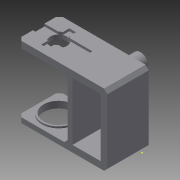
# Autodesk Inventor part: Pinza
Saved by Autodesk Inventor 2015 (Build 190159000, 159)
## iProperties
Created: 2013-10-22
Part Number: Pinza
Material: Genérico
Document SubType Name: Modeling
Designer: Gregorio
Density: 1 g/cm^3
Appearance: Valor por defecto
Author: Gregorio
Autodesk Inventor part; units mm, degrees
ref_plane "YZ Plane" through (0, 0, 0) normal (1, 0, 0) x (0, 1, 0)
ref_plane "XZ Plane" through (0, 0, 0) normal (0, 1, 0) x (-1, 0, 0)
ref_plane "XY Plane" through (0, 0, 0) normal (0, 0, 1) x (1, 0, 0)
sketch "Boceto1" plane through (0, 0, 0) normal (0, 1, 0) x (-1, 0, 0)
  line L0 (0, 0) -> (4, 0)
  line L1 (4, 0) -> (4, 43)
  line L2 (4, 43) -> (0, 43)
  line L3 (0, 43) -> (0, 0)
  line L4 (4, 43) -> (54, 43)
  line L5 (54, 43) -> (54, 39)
  line L6 (54, 39) -> (4, 39)
  line L7 (4, 39) -> (4, 43)
  line L8 (4, 0) -> (54, 0)
  line L9 (54, 0) -> (54, 4)
  line L10 (54, 4) -> (4, 4)
  line L11 (4, 4) -> (4, 0)
  dimension "d4" = 43
  dimension "d5" = 50
  dimension "d6" = 4
  dimension "d7" = 50
  dimension "d8" = 4
  dimension "d54" = 4
  constraints: 24 end point, 6 parallel, 3 horizontal, 3 perpendicular
  measures "d4" distance of L0.end L1.end
  measures "d5" distance of L5.end L6.end
  measures "d6" distance of L4.end L5.end
  measures "d7" distance of L10.end L9.end
  measures "d8" distance of L9.end L8.end
  measures "d54" distance of L1.end L2.end
extrude "Extrusión1" add sketch "Boceto1" along normal blind 25
sketch "Boceto3" plane through (-54, 0, 4) normal (0, 0, 1) x (1, 0, 0)
  line L0 (0, 0) -> (0, 25) projected
  circle A0 centre (12, 12.5) radius 9
  point P0 (54, 0)
  point P1 (0, 12.5)
  dimension "d19" = 18
  dimension "d20" = 12
  constraints: 1 centre point, 1 horizontal alignment, 1 midpoint
  measures "d19" diameter of A0
  measures "d20" distance from line of L0 A0.centre
extrude "Extrusión2" cut sketch "Boceto3" against normal blind 8 and the other way blind 2
sketch "Boceto8" plane through (-54, 0, 43) normal (0, 0, 1) x (1, 0, 0)
  circle A0 centre (12, 12.5) radius 5
  line L0 (0, 0) -> (0, 25) projected
  line L1 (0, 9) -> (0, 16)
  point P0 (0, 12.5)
  dimension "d40" = 10
  dimension "d42" = 12
  constraints: 2 end point, 1 centre point, 1 horizontal alignment, 1 midpoint, 1 point on line
  measures "d40" diameter of A0
  measures "d42" distance from line of L0 A0.centre
extrude "Extrusión7" cut sketch "Boceto8" against normal blind 5
sketch "Boceto9" plane through (-54, 0, 43) normal (0, 0, 1) x (1, 0, 0)
  circle A0 centre (12, 12.5) radius 5 projected
  line L0 (0, 16) -> (29, 16)
  line L1 (29, 16) -> (29, 9)
  line L2 (29, 9) -> (0, 9)
  line L3 (0, 9) -> (0, 16)
  dimension "d44" = 17
  dimension "d45" = 7
  constraints: 8 end point, 2 parallel, 1 horizontal, 1 perpendicular
  measures "d44" distance from line of L1 A0.centre
  measures "d45" distance of L0.end L1.end
sketch "Boceto10" plane through (-54, 0, 43) normal (0, 0, 1) x (1, 0, 0)
  circle A0 centre (12, 12.5) radius 5 projected
  line L0 (0, 0) -> (0, 25) projected
  line L1 (10, 21) -> (14, 21)
  line L2 (14, 21) -> (14, 4)
  line L3 (14, 4) -> (10, 4)
  line L4 (10, 4) -> (10, 21)
  point P0 (10, 12.5)
  point P1 (0, 12.5)
  point P2 (12, 21)
  dimension "d48" = 4
  dimension "d49" = 17
  constraints: 8 end point, 3 midpoint, 2 parallel, 1 horizontal, 1 horizontal alignment, 1 perpendicular, 1 vertical alignment
  measures "d48" distance of L1.start L1.end
  measures "d49" distance of L3.end L1.start
extrude "Extrusión8" cut sketch "Boceto10" against normal blind 1.5 contours L2 A0 L4 | A0 L4 L1 L2 | L2 L3 L4 A0
extrude "Extrusión9" cut sketch "Boceto9" against normal blind 1.5 contours A0 L2 L0 | A0 L0 L1 L2 | A0 L2 L3 L0
chamfer "Chaflán1" distance 2 angle 45 1 edges at (0, 12.5, 0)
chamfer "Chaflán2" distance 2 angle 45 1 edges at (0, 12.5, 43)
sketch "Boceto13" plane through (-54, 0, 4) normal (0, 0, 1) x (1, 0, 0)
  line L0 (0, 25) -> (50, 25) projected
  line L1 (29.9369, 25) -> (49.9369, 25)
  line L2 (49.9369, 25) -> (49.9369, 0)
  line L3 (49.9369, 0) -> (29.9369, 0)
  line L4 (29.9369, 0) -> (29.9369, 25)
  point P0 (54, 0)
  dimension "d80" = 20
  dimension "d81" = 25
  constraints: 8 end point, 2 parallel, 1 horizontal, 1 perpendicular, 1 point on line
  measures "d80" distance of L2.end L3.end
  measures "d81" distance of L3.end L1.start
extrude "Extrusión12" add sketch "Boceto13" along normal blind 5
sketch "Boceto14" plane through (-54, 0, 9) normal (0, 0, 1) x (1, 0, 0)
  line L0 (49.9369, 25) -> (32.9369, 25)
  line L1 (32.9369, 25) -> (32.9369, -5)
  line L2 (32.9369, -5) -> (49.9369, -5)
  line L3 (49.9369, -5) -> (49.9369, 25)
  dimension "d84" = 17
  dimension "d85" = 30
  constraints: 8 end point, 2 parallel, 1 horizontal, 1 perpendicular
  measures "d84" distance of L2.end L1.end
  measures "d85" distance of L1.end L0.end
extrude "Extrusión13" cut sketch "Boceto14" against normal blind 5
sketch "Boceto15" plane through (-4, 0, 4) normal (0, 0, 1) x (1, 0, 0)
  line L0 (0, 25) -> (0, 0) projected
  line L1 (-17.0631, 25) -> (0, 25)
  line L2 (0, 25) -> (0, 21)
  line L3 (0, 21) -> (-17.0631, 21)
  line L4 (-17.0631, 21) -> (-17.0631, 25)
  point P0 (4, 0)
  constraints: 8 end point, 2 parallel, 1 horizontal, 1 perpendicular, 1 point on line
extrude "Extrusión14" add sketch "Boceto15" along normal up to next
sketch "Boceto16" plane through (0, 25, 0) normal (0, 1, 0) x (1, 0, 0)
  circle A0 centre (-13, -15) radius 9
  line L0 (-21.0631, -4) -> (-4, -4) projected
  line L1 (-4, -39) -> (-4, -4) projected
  point P0 (0, 0)
  dimension "d90" = 11
  dimension "d91" = 18
  constraints: 1 centre point, 1 tangent
  measures "d90" distance from line of L0 A0.centre
  measures "d91" diameter of A0
extrude "Extrusión15" cut sketch "Boceto16" against normal blind 5
sketch "Boceto17" plane through (-4, 0, 39) normal (0, 0, -1) x (-1, 0, 0)
  line L0 (0, 0) -> (50, 0) projected
  line L1 (17.0631, 25) -> (20.0631, 25)
  line L2 (20.0631, 25) -> (20.0631, 0)
  line L3 (20.0631, 0) -> (17.0631, 0)
  line L4 (17.0631, 0) -> (17.0631, 25)
  point P0 (-4, 0)
  dimension "d94" = 3
  constraints: 8 end point, 2 parallel, 1 horizontal, 1 perpendicular, 1 point on line
  measures "d94" distance of L2.end L3.end
extrude "Extrusión16" add sketch "Boceto17" along normal up to next
sketch "Boceto18" plane through (0, 25, 0) normal (0, 1, 0) x (1, 0, 0)
  circle A0 centre (-13, -15) radius 9 projected
  line L0 (-54, -43) -> (-2, -43) projected
  circle A1 centre (-13, -35.3) radius 4.75
  point P0 (0, 0)
  dimension "d97" = 9.5
  dimension "d98" = 7.7
  constraints: 1 centre point, 1 vertical alignment
  measures "d97" diameter of A1
  measures "d98" distance from line of L0 A1.centre
extrude "Extrusión17" add sketch "Boceto18" along normal blind 8 contours A1
sketch "Boceto20" plane through (-21.0631, 21, 39) normal (0, -1, 0) x (1, 0, 0)
  arc A0 (17.0631, -24) -> (0, -20.0018) centre (8.0631, -24) ccw projected
  line L0 (0, -20.0018) -> (0, 0) projected
  line L1 (0, 0) -> (17.0631, 0)
  line L2 (17.0631, 0) -> (17.0631, -24)
  line L3 (17.0631, -24) -> (0, -24)
  line L4 (0, -24) -> (0, 0)
  point P0 (21.0631, -39)
  constraints: 8 end point, 2 parallel, 1 horizontal, 1 perpendicular
extrude "Extrusión19" add sketch "Boceto20" along normal blind 3 contours A0 L0 L1 L2
sketch "Boceto21" plane through (-21.0631, 18, 39) normal (0, -1, 0) x (1, 0, 0)
  arc A0 (17.0631, -24) -> (0, -20.0018) centre (8.0631, -24) ccw projected
  line L0 (1.9131, -30.2886) -> (14.2131, -30.2886)
  line L1 (14.2131, -30.2886) -> (14.2131, -6.6886)
  line L2 (14.2131, -6.6886) -> (1.9131, -6.6886)
  line L3 (1.9131, -6.6886) -> (1.9131, -30.2886)
  point P0 (21.0631, -39)
  point P1 (8.0631, -30.2886)
  dimension "d108" = 12.3
  dimension "d109" = 23.6
  constraints: 8 end point, 2 parallel, 1 horizontal, 1 midpoint, 1 perpendicular, 1 vertical alignment
  measures "d108" distance of L2.end L1.end
  measures "d109" distance of L1.end L0.end
extrude "Extrusión20" cut sketch "Boceto21" against normal blind 3
sketch "Boceto23" plane through (-54, 0, 4) normal (0, 0, 1) x (1, 0, 0)
  circle A0 centre (12, 12.5) radius 9 projected
  line L0 (29.9369, 0) -> (29.9369, 25) projected
  line L1 (0, 25) -> (29.9369, 25) projected
  line L2 (0, 0) -> (0, 25) projected
  line L3 (0, 0) -> (29.9369, 0) projected
  circle A1 centre (12, 12.5) radius 10
  point P0 (54, 0)
  dimension "d114" = 20
  constraints: 1 centre point, 1 coincident
  measures "d114" diameter of A1
extrude "Extrusión22" cut sketch "Boceto23" against normal blind 1 contours L3 L2 L1 L0
sketch "Boceto24" plane through (-13, 21, 4) normal (0, -1, 0) x (1, 0, 0)
  arc A0 (0, 0) -> (9, 11) centre (0, 9) ccw projected
  line L0 (9, 0) -> (-8.0631, 0) projected
  line L1 (9, 11) -> (9, 0) projected
  point P0 (13, -4)
  constraints: 1 other
sketch "Boceto25" plane through (-21.0631, 21, 4) normal (0, -1, 0) x (1, 0, 0)
  arc A0 (0, 7.0018) -> (17.0631, 11) centre (8.0631, 11) ccw projected
  line L0 (0, 0) -> (0, 7.0018) projected
  line L1 (17.0631, 0) -> (0, 0) projected
  point P0 (8.0631, 0)
  point P1 (21.0631, -4)
  constraints: 1 other
sketch "Boceto26" plane through (-21.0631, 21, 4) normal (0, -1, 0) x (1, 0, 0)
  arc A0 (0, 7.0018) -> (17.0631, 11) centre (8.0631, 11) ccw projected
  line L0 (0, 0) -> (0, 7.0018) projected
  line L1 (17.0631, 0) -> (0, 0) projected
  line L2 (17.0631, 11) -> (17.0631, 0) projected
  point P0 (21.0631, -4)
extrude "Extrusión25" add sketch "Boceto26" along normal blind 3
chamfer "Chaflán5" distance 2 angle 45 2 edges at (-24.0631, 12.5, 3) (-24.0631, 12.5, 39)
chamfer "Chaflán6" distance 2 angle 45 4 edges at (-54, 0, 41) (-54, 25, 41) (-54, 25, 1.5) (-54, 0, 1.5)
